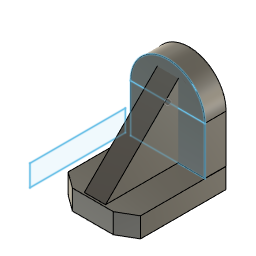
Model1 v1 (Autodesk Fusion 360 design; units mm, degrees)
Autodesk Fusion 360 part; units mm, degrees
sketch "Sketch1" plane through (0, 0, 0) normal (0, 1, 0) x (1, 0, 0)
  line L0 (15, -55) -> (57, -55)
  line L1 (57, -55) -> (57, -28)
  line L2 (57, -28) -> (15, -28)
  line L3 (15, -28) -> (15, -55)
  arc A0 (15, -55) -> (57, -55) centre (36, -55) ccw
  dimension "d1" = 42
  dimension "d2" = 27
  dimension "d3" = 42
  constraint horizontal L0
  constraint vertical L1
  constraint horizontal L2
  constraint vertical L3
  constraint midpoint L0 A0.centre
  measures "d1" distance of L0.start L0.end
  measures "d2" distance of L0.start L2.end
  measures "d3" diameter of A0
extrude "Extrude1" add sketch "Sketch1" along normal blind 12 makes body 1
sketch "Sketch2" plane through (0, 0, 0) normal (1, 0, 0) x (0, 1, 0)
  line L0 (11.9832, 27.9697) -> (-42.0168, 27.9697)
  line L1 (-42.0168, 27.9697) -> (-42.0168, 15.9697)
  line L2 (-42.0168, 15.9697) -> (11.9832, 15.9697)
  line L3 (11.9832, 15.9697) -> (11.9832, 27.9697)
  dimension "d6" = 54
  dimension "d7" = 12
  constraint horizontal L0
  constraint vertical L1
  constraint horizontal L2
  constraint vertical L3
  measures "d6" distance of L0.start L0.end
  measures "d7" distance of L0.start L2.end
extrude "Extrude2" add sketch "Sketch2" along normal blind 42 separate body makes body 2
move_face "MoveFace1" by (17.337, 0, -0.6971) 1 faces at (14, -6.0168, 27.9697) on bodies 2
move_body "Move1" bodies 2 to x (1, 0, 0) y (0, 1, 0) z (0, 0, 1) at (-0.024, 1.0073, -0.1439)
move_body "Move2" bodies 2 to x (1, 0, 0) y (0, 1, 0) z (0, 0, 1) at (14.8229, 0.3024, 0.2877)
move_body "Move3" bodies 2 to x (1, 0, 0) y (0, 1, 0) z (0, 0, 1) at (0.1298, -1.3016, 0.3922)
sketch "Sketch3" plane through (0, 0, 0) normal (1, 0, 0) x (0, 1, 0)
  line L0 (0, 28) -> (-42, 28)
  line L1 (-42, 28) -> (0, 70)
  line L2 (0, 70) -> (0, 28)
  constraint horizontal L0
  constraint perpendicular L0 L2
extrude "Extrude3" add sketch "Sketch3" along normal blind 12 separate body makes body 3
move_body "Move4" bodies 3 to x (1, 0, 0) y (0, 1, 0) z (0, 0, 1) at (30.8069, 0.0564, 0.1362)
move_body "Move5" bodies 3 to x (1, 0, 0) y (0, 1, 0) z (0, 0, 1) at (0, 0.8, 0)
move_body "Move6" bodies 3 to x (1, 0, 0) y (0, 1, 0) z (0, 0, 1) at (-0.9, 0, 0)
sketch "Sketch4" plane through (0, 0, 0) normal (0, 0, 1) x (1, 0, 0)
  line L0 (14.5054, -35.0252) -> (24.1764, -42.1296)
  line L1 (14.5054, -35.0252) -> (14.5054, -42.0056)
  line L2 (24.1764, -42.1296) -> (14.5054, -42.0056)
  line L3 (14.5054, -35.0252) -> (14.5054, -42.0056)
  dimension "d12" = 12
  constraint vertical L1
  constraint parallel L1 L3
  measures "d12" distance of L0.start L0.end
extrude "Extrude4" cut sketch "Sketch4" along normal blind 28 bodies 2
sketch "Sketch5" plane through (0, 0, 0) normal (0, 0, 1) x (1, 0, 0)
  line L0 (57.4466, -36.0522) -> (46.8956, -42.1773)
  line L1 (46.8956, -42.1773) -> (57.4466, -42.1773)
  line L2 (57.4466, -42.1773) -> (57.4466, -36.0522)
  dimension "d15" = 12.2
  constraint horizontal L1
  constraint perpendicular L1 L2
  measures "d15" distance of L0.start L0.end
extrude "Extrude5" cut sketch "Sketch5" along normal blind 31 bodies 2
